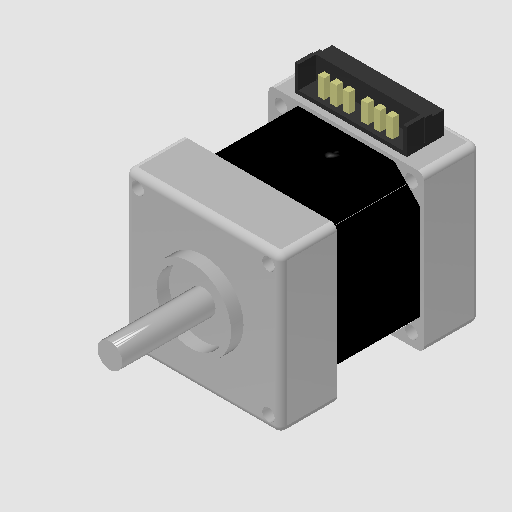
# Autodesk Inventor part: Part10
Saved by Autodesk Inventor 2017 (Build 210142000, 142)
## iProperties
Created: 2013-01-21
Part Number: Part10
Material: Generic
Document SubType Name: Modeling
Designer: despotis
Density: 1 g/cm^3
Appearance: Default
Author: despotis
Autodesk Inventor part; units mm, degrees
ref_plane "YZ Plane" through (0, 0, 0) normal (1, 0, 0) x (0, 1, 0)
sketch "Sketch1" plane through (0, 0, 0) normal (0, 0, 1) x (1, 0, 0)
  line L0 (0, 0) -> (12.5, 0)
  line L1 (12.5, 0) -> (12.5, 12.5)
  line L2 (12.5, 12.5) -> (0, 12.5)
  line L3 (0, 12.5) -> (0, 0)
  dimension "d0" = 12.5
  dimension "d2" = 12.5
  constraints: 8 end point, 2 parallel, 1 horizontal, 1 perpendicular
  measures "d0" distance of L1.end L2.end
  measures "d2" distance of L0.end L1.end
extrude "Extrusion1" add sketch "Sketch1" along normal blind 0.5
sketch "Sketch3" plane through (0, 0, 0.5) normal (0, 0, 1) x (1, 0, 0)
  line L0 (1.166, 12.2) -> (0.3, 11.2) projected
  line L1 (0.3, 11.2) -> (0.3, 1.3) projected
  line L2 (0.3, 1.3) -> (1.166, 0.3) projected
  line L3 (1.166, 0.3) -> (11.334, 0.3) projected
  line L4 (11.334, 0.3) -> (12.2, 1.3) projected
  line L5 (12.2, 1.3) -> (12.2, 11.2) projected
  line L6 (12.2, 11.2) -> (11.334, 12.2) projected
  line L7 (11.334, 12.2) -> (1.166, 12.2) projected
  line L8 (0.3, 11.2) -> (1.166, 12.2)
  line L9 (11.334, 12.2) -> (1.166, 12.2)
  line L10 (12.2, 11.2) -> (11.334, 12.2)
  line L11 (12.2, 11.2) -> (12.2, 1.3)
  line L12 (11.334, 0.3) -> (12.2, 1.3)
  line L13 (11.334, 0.3) -> (1.166, 0.3)
  line L14 (1.166, 0.3) -> (11.334, 0.3)
  line L15 (0, 0) -> (12.5, 0) projected
  line L16 (12.5, 0) -> (12.5, 12.5) projected
  line L17 (12.5, 12.5) -> (0, 12.5) projected
  line L18 (0, 12.5) -> (0, 0) projected
  constraints: 14 end point, 7 equal length
sketch "Sketch4" plane through (0, 0, 0.5) normal (0, 0, 1) x (1, 0, 0)
  line L0 (0, 0) -> (12.5, 0) projected
  line L1 (12.5, 0) -> (12.5, 12.5) projected
  line L2 (0, 12.5) -> (0, 0) projected
  line L3 (0, 0) -> (12.5, 0)
  line L4 (12.5, 0) -> (12.5, 12.5)
  line L5 (12.5, 12.5) -> (0, 12.5)
  line L6 (0, 12.5) -> (0, 0)
  line L7 (0, 0) -> (12.5, 0)
  line L8 (12.5, 0) -> (12.5, 12.5)
  line L9 (12.5, 12.5) -> (0, 12.5)
  line L10 (0, 12.5) -> (0, 0)
  circle A0 centre (1.0102, 0.9893) radius 0.5
  line L11 (1.3674, 1.3391) -> (2.385, 0.3)
  line L12 (1.3674, 1.3391) -> (0.3, 2.4291)
  circle A1 centre (11.4898, 0.9893) radius 0.5
  line L13 (11.1326, 1.3391) -> (10.115, 0.3)
  line L14 (11.1326, 1.3391) -> (12.2, 2.4291)
  circle A2 centre (1.0102, 11.5107) radius 0.5
  line L15 (1.3674, 11.1609) -> (2.385, 12.2)
  line L16 (1.3674, 11.1609) -> (0.3, 10.0709)
  line L17 (11.1326, 11.1609) -> (12.2, 10.0709)
  line L18 (11.1326, 11.1609) -> (10.115, 12.2)
  circle A3 centre (11.4898, 11.5107) radius 0.5
  line L19 (2.385, 0.3) -> (10.115, 0.3)
  line L20 (12.2, 2.4291) -> (12.2, 10.0709)
  line L21 (10.115, 12.2) -> (2.385, 12.2)
  line L22 (0.3, 10.0709) -> (0.3, 2.4291)
  dimension "d21" = 1
  dimension "d22" = 0.3
  dimension "d23" = 0.3
  dimension "d24" = 0.3
  dimension "d25" = 0.3
  constraints: 40 end point, 6 parallel, 3 horizontal, 3 perpendicular, 1 collinear, 13 other
  measures "d22" distance between parallel lines of L5 L21
  measures "d23" distance between parallel lines of L1 L20
  measures "d24" distance between parallel lines of L0 L19
  measures "d25" distance between parallel lines of L2 L22
extrude "Extrusion3" add sketch "Sketch4" along normal blind 4
sketch "Sketch5" plane through (0, 0, 4.5) normal (0, 0, 1) x (1, 0, 0)
  circle A0 centre (1.0102, 0.9893) radius 0.5 projected
  line L0 (1.3674, 1.3391) -> (0.3, 2.4291) projected
  line L1 (0.3, 2.4291) -> (0.3, 10.0709) projected
  line L2 (0.3, 10.0709) -> (1.3674, 11.1609) projected
  circle A1 centre (1.0102, 11.5107) radius 0.5 projected
  line L3 (1.3674, 11.1609) -> (2.385, 12.2) projected
  line L4 (2.385, 12.2) -> (10.115, 12.2) projected
  line L5 (10.115, 12.2) -> (11.1326, 11.1609) projected
  circle A2 centre (11.4898, 11.5107) radius 0.5 projected
  line L6 (11.1326, 11.1609) -> (12.2, 10.0709) projected
  line L7 (12.2, 10.0709) -> (12.2, 2.4291) projected
  line L8 (12.2, 2.4291) -> (11.1326, 1.3391) projected
  circle A3 centre (11.4898, 0.9893) radius 0.5 projected
  line L9 (11.1326, 1.3391) -> (10.115, 0.3) projected
  line L10 (10.115, 0.3) -> (2.385, 0.3) projected
  line L11 (2.385, 0.3) -> (1.3674, 1.3391) projected
  line L12 (0.3, 10.0709) -> (2.385, 12.2)
  line L13 (2.385, 12.2) -> (10.115, 12.2)
  line L14 (10.115, 12.2) -> (12.2, 10.0709)
  line L15 (12.2, 10.0709) -> (12.2, 2.4291)
  line L16 (12.2, 2.4291) -> (10.115, 0.3)
  line L17 (10.115, 0.3) -> (2.385, 0.3)
  line L18 (2.385, 0.3) -> (0.3, 2.4291)
  line L19 (0.3, 2.4291) -> (0.3, 10.0709)
  constraints: 16 end point, 4 other
extrude "Extrusion4" add sketch "Sketch5" against normal blind 4 and the other way blind 3.5 contours L0 L1 L2 L3 L4 L5 L6 L7 L8 L9 L10 L11
ref_plane "Work Plane1" through (0, 0, 8) normal (0, 0, 1) x (1, 0, 0)
sketch "Sketch6" plane through (0, 0, 8) normal (0, 0, 1) x (1, 0, 0)
  point P0 (0, 0)
fillet "Fillet1" radius 0.5 8 edges at (12.5, 12.5, 2.25) (6.25, 12.5, 0) (0, 12.5, 2.25) (12.5, 0, 2.25) (12.5, 6.25, 0) (6.25, 0, 0) (0, 6.25, 0) (0, 0, 2.25)
mirror "Mirror1" about plane through (0, 0, 8) normal (0, 0, 1) of "Extrusion1"
mirror "Mirror2" about plane through (0, 0, 8) normal (0, 0, 1) of "Extrusion3"
mirror "Mirror3" about plane through (0, 0, 8) normal (0, 0, 1) of "Extrusion4"
sketch "Sketch7" plane through (0, 0, 16) normal (0, 0, 1) x (1, 0, 0)
  circle A0 centre (1, 1) radius 0.5
  circle A1 centre (11.5, 1) radius 0.5
  circle A2 centre (11.5, 11.5) radius 0.5
  circle A3 centre (1, 11.5) radius 0.5
  dimension "d34" = 1
  dimension "d35" = 1
  dimension "d36" = 1
  dimension "d37" = 1
  constraints: 4 centre point
  measures "d34" diameter of A0
  measures "d35" diameter of A1
  measures "d36" diameter of A2
  measures "d37" diameter of A3
hole "Hole1" at (1, 11.5, 16) at (11.5, 11.5, 16) at (1, 1, 16) at (11.5, 1, 16) direction (0, 0, -1) diameter 1 end through all
fillet "Fillet2" radius 0.5 8 edges at (0, 12.5, 13.75) (6.25, 12.5, 16) (12.5, 12.5, 13.75) (12.5, 6.25, 16) (0, 6.25, 16) (6.25, 0, 16) (12.5, 0, 13.75) (0, 0, 13.75)
sketch "Sketch8" plane through (1, 12, 16) normal (0, 0, 1) x (1, 0, 0)
  circle A0 centre (5.25, -5.75) radius 1
  point P0 (-1, -12)
  dimension "d46" = 2
  constraints: 1 centre point
  measures "d46" diameter of A0
hole "Hole2" at (6.25, 6.25, 16) direction (0, 0, -1) diameter 2 depth 0.5
sketch "Sketch9" plane through (6.25, 6.25, 15.5) normal (0, 0, 1) x (1, 0, 0)
  circle A0 centre (0, 0) radius 1 projected
  circle A1 centre (0, 0) radius 1
  point P0 (-6.25, -6.25)
  dimension "d56" = 2
  constraints: 1 centre point
  measures "d56" diameter of A1
extrude "Extrusion5" add sketch "Sketch9" along normal blind 8
sketch "Sketch10" plane through (1, 12, 16) normal (0, 0, 1) x (1, 0, 0)
  circle A0 centre (5.25, -5.75) radius 3.25
  circle A1 centre (5.25, -5.75) radius 2.75
  point P0 (-1, -12)
  dimension "d59" = 6.5
  dimension "d60" = 5.5
  constraints: 2 centre point
  measures "d59" diameter of A0
  measures "d60" diameter of A1
extrude "Extrusion6" add sketch "Sketch10" along normal blind 1
sketch "Sketch11" plane through (0.5, 12.5, 0.5) normal (0, 1, 0) x (1, 0, 0)
  line L0 (1.1263, -0.5124) -> (10.1263, -0.5124)
  line L1 (10.1263, -0.5124) -> (10.1263, -3.5124)
  line L2 (10.1263, -3.5124) -> (1.1263, -3.5124)
  line L3 (1.1263, -3.5124) -> (1.1263, -0.5124)
  point P0 (-0.5, 0.5)
  dimension "d63" = 9
  dimension "d64" = 3
  constraints: 8 end point, 2 parallel, 1 horizontal, 1 perpendicular
  measures "d63" distance of L1.end L2.end
  measures "d64" distance of L0.end L1.end
extrude "Extrusion7" add sketch "Sketch11" along normal blind 0.3
ref_plane "Work Plane2" through (0.4997, 12.8, 1.6376) normal (0, 1, 0) x (1, 0, 0)
sketch "Sketch12" plane through (0.4997, 12.8, 1.6376) normal (0, 1, 0) x (1, 0, 0)
  line L0 (2.6263, -2.0124) -> (3.1263, -2.0124)
  line L1 (3.1263, -2.0124) -> (3.1263, -1.5124)
  line L2 (3.1263, -1.5124) -> (2.6263, -1.5124)
  line L3 (2.6263, -1.5124) -> (2.6263, -2.0124)
  line L4 (4.1263, -2.0124) -> (3.6263, -2.0124)
  line L5 (3.6263, -2.0124) -> (3.6263, -1.5124)
  line L6 (3.6263, -1.5124) -> (4.1263, -1.5124)
  line L7 (4.1263, -1.5124) -> (4.1263, -2.0124)
  line L8 (4.6263, -2.0124) -> (5.1263, -2.0124)
  line L9 (5.1263, -2.0124) -> (5.1263, -1.5124)
  line L10 (5.1263, -1.5124) -> (4.6263, -1.5124)
  line L11 (4.6263, -1.5124) -> (4.6263, -2.0124)
  line L12 (8.6263, -2.0124) -> (8.1263, -2.0124)
  line L13 (8.1263, -2.0124) -> (8.1263, -1.5124)
  line L14 (8.1263, -1.5124) -> (8.6263, -1.5124)
  line L15 (8.6263, -1.5124) -> (8.6263, -2.0124)
  line L16 (7.1263, -2.0124) -> (7.6263, -2.0124)
  line L17 (7.6263, -2.0124) -> (7.6263, -1.5124)
  line L18 (7.6263, -1.5124) -> (7.1263, -1.5124)
  line L19 (7.1263, -1.5124) -> (7.1263, -2.0124)
  line L20 (6.6263, -2.0124) -> (6.1263, -2.0124)
  line L21 (6.1263, -2.0124) -> (6.1263, -1.5124)
  line L22 (6.1263, -1.5124) -> (6.6263, -1.5124)
  line L23 (6.6263, -1.5124) -> (6.6263, -2.0124)
  point P0 (-0.5, 0.5)
  constraints: 48 end point, 6 parallel, 3 horizontal, 3 perpendicular
extrude "Extrusion8" add sketch "Sketch12" along normal blind 1.5
sketch "Sketch13" plane through (0.5, 12.8, 0.5) normal (0, 1, 0) x (1, 0, 0)
  line L0 (1.1263, -2.0124) -> (10.1263, -2.0124)
  line L1 (10.1263, -2.0124) -> (10.1263, -0.5124)
  line L2 (10.1263, -0.5124) -> (1.1263, -0.5124)
  line L3 (1.1263, -0.5124) -> (1.1263, -2.0124)
  point P0 (-0.5, 0.5)
  constraints: 8 end point, 2 parallel, 1 horizontal, 1 perpendicular
extrude "Extrusion9" add sketch "Sketch13" along normal blind 1.5
sketch "Sketch14" plane through (0.5, 14.3, 0.5) normal (0, 1, 0) x (1, 0, 0)
  line L0 (1.1263, -2.0124) -> (10.1263, -2.0124)
  line L1 (10.1263, -2.0124) -> (10.1263, -1.5124)
  line L2 (10.1263, -1.5124) -> (1.1263, -1.5124)
  line L3 (1.1263, -1.5124) -> (1.1263, -2.0124)
  point P0 (-0.5, 0.5)
  dimension "d81" = 0.5
  constraints: 8 end point, 2 parallel, 1 horizontal, 1 perpendicular
  measures "d81" distance of L1.end L0.end
extrude "Extrusion10" add sketch "Sketch14" along normal blind 0.2
sketch "Sketch15" plane through (0.5, 12.8, 0.5) normal (0, 1, 0) x (1, 0, 0)
  line L0 (1.1263, -3.5124) -> (1.4263, -3.5124)
  line L1 (1.4263, -3.5124) -> (1.4263, -2.1124)
  line L2 (1.4263, -2.1124) -> (1.1263, -2.1124)
  line L3 (1.1263, -2.1124) -> (1.1263, -3.5124)
  line L4 (10.1263, -3.5124) -> (9.8263, -3.5124)
  line L5 (9.8263, -3.5124) -> (9.8263, -2.1124)
  line L6 (9.8263, -2.1124) -> (10.1263, -2.1124)
  line L7 (10.1263, -2.1124) -> (10.1263, -3.5124)
  point P0 (-0.5, 0.5)
  dimension "d84" = 0.3
  dimension "d85" = 1.4
  dimension "d86" = 0.3
  constraints: 16 end point, 4 parallel, 2 horizontal, 2 perpendicular
  measures "d84" distance of L2.end L1.end
  measures "d85" distance of L1.end L0.end
  measures "d86" distance of L5.end L6.end
extrude "Extrusion11" add sketch "Sketch15" along normal blind 1.8
body "Solid1"
